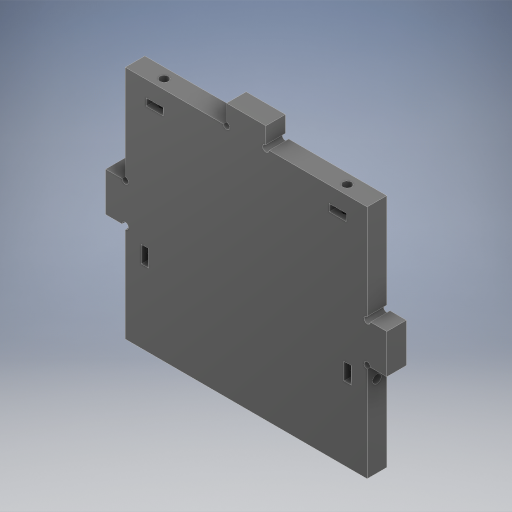
# Autodesk Inventor part: overhead
Saved by Autodesk Inventor 2024 (Build 280153000, 153)
## iProperties
Created: 2024-09-05
Part Number: overhead
Material: PMMA 플라스틱
Document SubType Name: Modeling
Designer: msi
Density: 1.188 g/cm^3
Appearance: 매끄러움 - 검은색
Author: msi
Autodesk Inventor part; units mm, degrees
ref_plane "YZ Plane" through (0, 0, 0) normal (1, 0, 0) x (0, 1, 0)
ref_plane "XZ Plane" through (0, 0, 0) normal (0, 1, 0) x (-1, 0, 0)
ref_plane "XY Plane" through (0, 0, 0) normal (0, 0, 1) x (1, 0, 0)
sketch "스케치1" plane through (0, 0, 0) normal (0, 0, 1) x (1, 0, 0)
  line L0 (-6.05, -3) -> (-6.05, 3) projected
  line L1 (6.05, -3) -> (-6.05, -3) projected
  line L2 (6.05, 3) -> (6.05, -3) projected
  line L3 (-6.05, 3) -> (6.05, 3) projected
  line L4 (6.05, 3) -> (6.05, -3) projected
  line L5 (6.05, -3) -> (43, -3) projected
  line L6 (43, 3) -> (43, -3) projected
  line L7 (6.05, 3) -> (43, 3) projected
  circle A0 centre (20, 0) radius 1.35 projected
  circle A1 centre (-20, 0) radius 1.35 projected
  line L8 (-6.05, -3) -> (-6.05, 3) projected
  line L9 (-6.05, 3) -> (-43, 3) projected
  line L10 (-43, -3) -> (-43, 3) projected
  line L11 (-6.05, -3) -> (-43, -3) projected
  line L12 (-43, -32.95) -> (-37, -32.95) projected
  line L13 (-37, -32.95) -> (-37, -3) projected
  line L14 (-37, -3) -> (-43, -3) projected
  line L15 (-43, -3) -> (-43, -32.95) projected
  line L16 (-43, -45.05) -> (-43, -32.95) projected
  line L17 (-37, -45.05) -> (-43, -45.05) projected
  line L18 (-37, -32.95) -> (-37, -45.05) projected
  line L19 (-43, -32.95) -> (-37, -32.95) projected
  line L20 (-37, -45.05) -> (-43, -45.05) projected
  line L21 (-43, -45.05) -> (-43, -75) projected
  line L22 (-43, -75) -> (-37, -75) projected
  line L23 (-37, -75) -> (-37, -45.05) projected
  line L24 (37, -32.95) -> (43, -32.95) projected
  line L25 (43, -32.95) -> (43, -3) projected
  line L26 (43, -3) -> (37, -3) projected
  line L27 (37, -3) -> (37, -32.95) projected
  line L28 (37, -45.05) -> (37, -32.95) projected
  line L29 (43, -45.05) -> (37, -45.05) projected
  line L30 (43, -32.95) -> (43, -45.05) projected
  line L31 (37, -32.95) -> (43, -32.95) projected
  line L32 (43, -45.05) -> (37, -45.05) projected
  line L33 (37, -45.05) -> (37, -75) projected
  line L34 (37, -75) -> (43, -75) projected
  line L35 (43, -75) -> (43, -45.05) projected
  line L36 (-37, -3) -> (37, -3)
  line L37 (37, -3) -> (37, -75)
  line L38 (37, -75) -> (-37, -75)
  line L39 (-37, -75) -> (-37, -3)
  line L40 (6, -3) -> (-6, -3)
  line L41 (-6, -3) -> (-6, 3)
  line L42 (-6, 3) -> (6, 3)
  line L43 (6, 3) -> (6, -3)
  line L44 (37, -33) -> (43, -33)
  line L45 (43, -33) -> (43, -45)
  line L46 (43, -45) -> (37, -45)
  line L47 (37, -45) -> (37, -33)
  line L48 (-37, -33) -> (-43, -33)
  line L49 (-43, -33) -> (-43, -45)
  line L50 (-43, -45) -> (-37, -45)
  line L51 (-37, -45) -> (-37, -33)
  point P0 (0, 0)
  dimension "d0" = 12
  dimension "d1" = 6
  dimension "d2" = 6
  dimension "d3" = 12
  dimension "d4" = 6
  dimension "d5" = 12
  constraints: 32 end point, 8 parallel, 4 horizontal, 4 perpendicular, 3 point on line
  measures "d0" distance of L41.end L42.end
  measures "d1" distance of L40.end L41.end
  measures "d2" distance of L45.end L46.end
  measures "d3" distance of L44.end L45.end
  measures "d4" distance of L50.end L49.end
  measures "d5" distance of L49.end L48.end
extrude "돌출1" add sketch "스케치1" along normal blind 6 contours L1 L5 L27 L28 L33 L38 L23 L18 L13 L11 | L41 L3 L43 L1 | L18 L50 L16 L48 | L44 L30 L46 L28
sketch "스케치2" plane through (-6, 3, 0) normal (0, 1, 0) x (1, 0, 0)
  circle A0 centre (34, -3.1) radius 1.35 projected
  circle A1 centre (-22, -3.1) radius 1.35 projected
  circle A2 centre (34, -3.1) radius 1.35
  circle A3 centre (-22, -3.1) radius 1.35
  point P0 (6, 0)
  constraints: 2 centre point, 2 coincident, 2 concentric
extrude "돌출2" cut sketch "스케치2" against normal blind 20
sketch "스케치3" plane through (-43, -45, 0) normal (-1, 0, 0) x (0, 0, 1)
  circle A0 centre (3.1, -5.05) radius 1.35 projected
  circle A1 centre (3.1, -5.05) radius 1.35
  point P0 (0, 45)
  constraints: 1 centre point, 1 coincident, 1 concentric
extrude "돌출3" cut sketch "스케치3" against normal blind 20
sketch "스케치4" plane through (43, -45, 0) normal (1, 0, 0) x (0, 0, -1)
  circle A0 centre (-3, -5.05) radius 1.35 projected
  circle A1 centre (-3, -5.05) radius 1.35
  point P0 (0, 45)
  constraints: 1 centre point, 1 coincident, 1 concentric
extrude "돌출4" cut sketch "스케치4" against normal blind 20
sketch "스케치5" plane through (0, 0, 6) normal (0, 0, 1) x (1, 0, 0)
  line L0 (37, -48.7) -> (23, -48.7) projected
  line L1 (37, -51.4) -> (23, -51.4) projected
  line L2 (-37, -51.4) -> (-23, -51.4) projected
  line L3 (-37, -48.7) -> (-23, -48.7) projected
  line L4 (-26.65, -3) -> (-26.65, -17) projected
  line L5 (-29.35, -3) -> (-29.35, -17) projected
  line L6 (29.35, -3) -> (29.35, -17) projected
  line L7 (26.65, -3) -> (26.65, -17) projected
  line L8 (31, -51.4) -> (31, -48.7)
  line L9 (-31, -51.4) -> (-31, -48.7)
  line L10 (29.35, -9) -> (26.65, -9)
  line L11 (-26.65, -9) -> (-29.35, -9)
  line L12 (25.4, -7.9) -> (30.6, -7.9)
  line L13 (30.6, -7.9) -> (30.6, -10.1)
  line L14 (30.6, -10.1) -> (25.4, -10.1)
  line L15 (25.4, -10.1) -> (25.4, -7.9)
  line L16 (25.4, -7.9) -> (30.6, -10.1) construction
  line L17 (30.6, -7.9) -> (25.4, -10.1) construction
  line L18 (29.9, -47.45) -> (32.1, -47.45)
  line L19 (32.1, -47.45) -> (32.1, -52.65)
  line L20 (32.1, -52.65) -> (29.9, -52.65)
  line L21 (29.9, -52.65) -> (29.9, -47.45)
  line L22 (29.9, -47.45) -> (32.1, -52.65) construction
  line L23 (32.1, -47.45) -> (29.9, -52.65) construction
  line L24 (-30.6, -7.9) -> (-25.4, -7.9)
  line L25 (-25.4, -7.9) -> (-25.4, -10.1)
  line L26 (-25.4, -10.1) -> (-30.6, -10.1)
  line L27 (-30.6, -10.1) -> (-30.6, -7.9)
  line L28 (-30.6, -7.9) -> (-25.4, -10.1) construction
  line L29 (-25.4, -7.9) -> (-30.6, -10.1) construction
  line L30 (-32.1, -47.45) -> (-29.9, -47.45)
  line L31 (-29.9, -47.45) -> (-29.9, -52.65)
  line L32 (-29.9, -52.65) -> (-32.1, -52.65)
  line L33 (-32.1, -52.65) -> (-32.1, -47.45)
  line L34 (-32.1, -47.45) -> (-29.9, -52.65) construction
  line L35 (-29.9, -47.45) -> (-32.1, -52.65) construction
  point P0 (0, 0)
  point P1 (28, -9)
  point P2 (31, -50.05)
  point P3 (-28, -9)
  point P4 (-31, -50.05)
  dimension "d14" = 5.2
  dimension "d15" = 2.2
  dimension "d16" = 2.2
  dimension "d17" = 5.2
  dimension "d18" = 5.2
  dimension "d19" = 2.2
  dimension "d20" = 2.2
  dimension "d21" = 5.2
  constraints: 56 end point, 12 midpoint, 8 parallel, 8 point on line, 7 perpendicular, 4 horizontal, 1 vertical
  measures "d14" distance of L13.end L14.end
  measures "d15" distance of L12.end L13.end
  measures "d16" distance of L19.end L20.end
  measures "d17" distance of L18.end L19.end
  measures "d18" distance of L25.end L26.end
  measures "d19" distance of L24.end L25.end
  measures "d20" distance of L31.end L32.end
  measures "d21" distance of L30.end L31.end
extrude "돌출5" cut sketch "스케치5" against normal blind 20
sketch "스케치6" plane through (0, 0, 6) normal (0, 0, 1) x (1, 0, 0)
  line L0 (-32.1, -52.65) -> (-32.1, -47.45) projected
  line L1 (-32.1, -47.45) -> (-29.9, -47.45) projected
  line L2 (-29.9, -47.45) -> (-29.9, -52.65) projected
  line L3 (-29.9, -52.65) -> (-32.1, -52.65) projected
  line L4 (29.9, -52.65) -> (29.9, -47.45) projected
  line L5 (29.9, -47.45) -> (32.1, -47.45) projected
  line L6 (32.1, -47.45) -> (32.1, -52.65) projected
  line L7 (32.1, -52.65) -> (29.9, -52.65) projected
  line L8 (-30.6, -7.9) -> (-25.4, -7.9) projected
  line L9 (-25.4, -7.9) -> (-25.4, -10.1) projected
  line L10 (-25.4, -10.1) -> (-30.6, -10.1) projected
  line L11 (-30.6, -10.1) -> (-30.6, -7.9) projected
  line L12 (30.6, -10.1) -> (25.4, -10.1) projected
  line L13 (25.4, -10.1) -> (25.4, -7.9) projected
  line L14 (25.4, -7.9) -> (30.6, -7.9) projected
  line L15 (30.6, -7.9) -> (30.6, -10.1) projected
  line L16 (37, -75) -> (37, -45) projected
  line L17 (37, -45) -> (43, -45) projected
  line L18 (43, -45) -> (43, -33) projected
  line L19 (43, -33) -> (37, -33) projected
  line L20 (37, -33) -> (37, -3) projected
  line L21 (37, -3) -> (6, -3) projected
  line L22 (6, -3) -> (6, 3) projected
  line L23 (6, 3) -> (-6, 3) projected
  line L24 (-6, 3) -> (-6, -3) projected
  line L25 (-6, -3) -> (-37, -3) projected
  line L26 (-37, -3) -> (-37, -33) projected
  line L27 (-37, -33) -> (-43, -33) projected
  line L28 (-43, -33) -> (-43, -45) projected
  line L29 (-43, -45) -> (-37, -45) projected
  line L30 (-37, -45) -> (-37, -75) projected
  line L31 (-37, -75) -> (37, -75) projected
  circle A0 centre (6, -3) radius 1
  circle A1 centre (-6, -3) radius 1
  circle A2 centre (37, -33) radius 1
  circle A3 centre (37, -45) radius 1
  circle A4 centre (-37, -33) radius 1
  circle A5 centre (-37, -45) radius 1
  point P0 (0, 0)
  point P1 (38, -45)
  point P2 (37, -46)
  point P3 (-37, -46)
  point P4 (-38, -45)
  point P5 (6, -2)
  point P6 (7, -3)
  dimension "d24" = 2
  dimension "d25" = 2
  dimension "d26" = 2
  dimension "d27" = 2
  dimension "d28" = 2
  dimension "d29" = 2
  constraints: 6 centre point, 6 coincident
  measures "d24" diameter of A0
  measures "d25" diameter of A1
  measures "d26" diameter of A2
  measures "d27" diameter of A3
  measures "d28" diameter of A4
  measures "d29" diameter of A5
extrude "돌출6" cut sketch "스케치6" against normal through all contours A3 L17 L16 | L30 L29 A5 | A2 L20 L19 | L19 L20 A2 | A4 L26 L27 | L27 L26 A4 | A0 L22 L21 | A1 L24 L25 | L25 L24 A1 picked at (36.339, -44.9727) picked at (-37.1584, -44.3574) picked at (5.6614, -3.5683)
